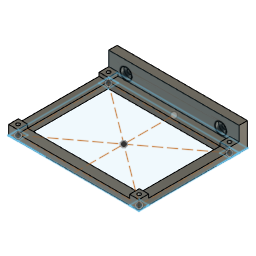
soporteSKR v3 (Autodesk Fusion 360 design; units mm, degrees)
Autodesk Fusion 360 part; units mm, degrees
sketch "Sketch7" plane through (0, 0, 0) normal (0, 0, 1) x (1, 0, 0)
  line L0 (9.0135, 7.5242) -> (118.6835, 7.5242)
  line L1 (118.6835, 7.5242) -> (118.6835, 98.8242)
  line L2 (118.6835, 98.8242) -> (9.0135, 98.8242)
  line L3 (9.0135, 98.8242) -> (9.0135, 7.5242)
  line L4 (63.8485, 7.5242) -> (63.8485, 91.8242) construction
  line L5 (118.6835, 91.8242) -> (9.0135, 91.8242)
  line L6 (12.9235, 11.6242) -> (114.7735, 11.6242) construction
  line L7 (114.7735, 11.6242) -> (114.7735, 87.7242) construction
  line L8 (114.7735, 87.7242) -> (12.9235, 87.7242) construction
  line L9 (12.9235, 87.7242) -> (12.9235, 11.6242) construction
  line L10 (12.9235, 11.6242) -> (114.7735, 87.7242) construction
  line L11 (114.7735, 11.6242) -> (12.9235, 87.7242) construction
  line L12 (9.0135, 91.8242) -> (16.8335, 91.8242)
  line L13 (16.8335, 91.8242) -> (16.8335, 83.6242)
  line L14 (16.8335, 83.6242) -> (9.0135, 83.6242)
  line L15 (9.0135, 83.6242) -> (9.0135, 91.8242)
  line L16 (9.0135, 91.8242) -> (16.8335, 83.6242) construction
  line L17 (16.8335, 91.8242) -> (9.0135, 83.6242) construction
  line L18 (9.0135, 7.5242) -> (16.8335, 7.5242)
  line L19 (16.8335, 7.5242) -> (16.8335, 15.7242)
  line L20 (16.8335, 15.7242) -> (9.0135, 15.7242)
  line L21 (9.0135, 15.7242) -> (9.0135, 7.5242)
  line L22 (9.0135, 7.5242) -> (16.8335, 15.7242) construction
  line L23 (16.8335, 7.5242) -> (9.0135, 15.7242) construction
  line L24 (118.6835, 7.5242) -> (110.8635, 7.5242)
  line L25 (110.8635, 7.5242) -> (110.8635, 15.7242)
  line L26 (110.8635, 15.7242) -> (118.6835, 15.7242)
  line L27 (118.6835, 15.7242) -> (118.6835, 7.5242)
  line L28 (118.6835, 7.5242) -> (110.8635, 15.7242) construction
  line L29 (110.8635, 7.5242) -> (118.6835, 15.7242) construction
  line L30 (118.6835, 91.8242) -> (110.8635, 91.8242)
  line L31 (110.8635, 91.8242) -> (110.8635, 83.6242)
  line L32 (110.8635, 83.6242) -> (118.6835, 83.6242)
  line L33 (118.6835, 83.6242) -> (118.6835, 91.8242)
  line L34 (118.6835, 91.8242) -> (110.8635, 83.6242) construction
  line L35 (110.8635, 91.8242) -> (118.6835, 83.6242) construction
  circle A0 centre (12.9235, 87.7242) radius 1.5
  circle A1 centre (114.7735, 87.7242) radius 1.5
  circle A2 centre (12.9235, 11.6242) radius 1.5
  circle A3 centre (114.7735, 11.6242) radius 1.5
  point P0 (63.8485, 49.6742)
  point P1 (12.9235, 87.7242)
  point P2 (12.9235, 11.6242)
  point P3 (114.7735, 11.6242)
  point P4 (114.7735, 87.7242)
  dimension "d70" = 109.67
  dimension "d71" = 91.3
  dimension "d72" = 84.3
  dimension "d73" = 101.85
  dimension "d74" = 76.1
  dimension "d89" = 3
  dimension "d90" = 3
  dimension "d91" = 3
  dimension "d92" = 3
  constraint horizontal L0
  constraint vertical L1
  constraint horizontal L2
  constraint vertical L3
  constraint midpoint L0 L4.start
  constraint perpendicular L0 L4
  constraint coincident L1 L5.start
  constraint coincident L3 L5.end
  constraint perpendicular L3 L5
  constraint horizontal L6
  constraint perpendicular L6 L7
  constraint parallel L6 L8
  constraint parallel L7 L9
  constraint coincident L10 P0
  constraint coincident L11 P0
  constraint midpoint L4 P0
  constraint horizontal L12
  constraint perpendicular L12 L13
  constraint parallel L12 L14
  constraint parallel L13 L15
  constraint coincident L16 P1
  constraint coincident L17 P1
  constraint coincident P1 L8.end
  constraint horizontal L18
  constraint perpendicular L18 L19
  constraint parallel L18 L20
  constraint parallel L19 L21
  constraint coincident L22 P2
  constraint coincident L23 P2
  constraint coincident P2 L6.start
  constraint horizontal L24
  constraint perpendicular L24 L25
  constraint parallel L24 L26
  constraint parallel L25 L27
  constraint coincident L28 P3
  constraint coincident L29 P3
  constraint coincident P3 L6.end
  constraint horizontal L30
  constraint perpendicular L30 L31
  constraint parallel L30 L32
  constraint parallel L31 L33
  constraint coincident L34 P4
  constraint coincident L35 P4
  constraint coincident P4 L7.end
  measures "d70" distance of L0.start L0.end
  measures "d71" distance of L0.start L2.end
  measures "d72" distance of L4.start L4.end
  measures "d73" distance of P4 P1
  measures "d74" distance of P3 P4
  measures "d89" diameter of A0
  measures "d90" diameter of A1
  measures "d91" diameter of A2
  measures "d92" diameter of A3
extrude "Extrude11" add sketch "Sketch7" along normal blind 5 contours L0 L3 L18 L19 L20 L21 | L0 L1 L3 L5 L13 L14 L19 L20 L25 L26 L31 L32 | L0 L1 L24 L25 L26 L27 | L3 L5 L12 L13 L14 L15 | L1 L5 L30 L31 L32 L33 | A0 | A1 | A2 | A3
extrude "Extrude13" cut sketch "Sketch7" along normal blind 8 contours L0 L3 L18 L19 L20 L21 | L0 L1 L24 L25 L26 L27 | L3 L5 L12 L13 L14 L15 | L1 L5 L30 L31 L32 L33 | A0 | A1 | A2 | A3
extrude "Extrude14" add sketch "Sketch7" along normal blind 8 contours L0 L3 L18 L19 L20 L21 | L0 L1 L24 L25 L26 L27 | L3 L5 L12 L13 L14 L15 | L1 L5 L30 L31 L32 L33 | A0 | A1 | A2 | A3
extrude "Extrude15" add sketch "Sketch7" along normal blind 20 contours L1 L2 L3 L5 L12 L30
extrude "Extrude16" cut sketch "Sketch7" along normal blind 22 contours A0 | A1 | A2 | A3
hole "Hole8" at (103.6835, 91.8242, 14) at (24.0135, 91.8242, 14) direction (0, 1, 0) diameter 4 end through all
sketch "Sketch10" plane through (0, 0, 5) normal (0, 0, 1) x (-1, 0, 0)
  line L0 (-16.8335, -83.6242) -> (-9.0135, -83.6242)
  line L1 (-9.0135, -83.6242) -> (-9.0135, -15.7242)
  line L2 (-9.0135, -15.7242) -> (-16.8335, -15.7242)
  line L3 (-16.8335, -15.7242) -> (-16.8335, -7.5242)
  line L4 (-16.8335, -7.5242) -> (-110.8635, -7.5242)
  line L5 (-110.8635, -7.5242) -> (-110.8635, -15.7242)
  line L6 (-110.8635, -15.7242) -> (-118.6835, -15.7242)
  line L7 (-118.6835, -15.7242) -> (-118.6835, -83.6242)
  line L8 (-118.6835, -83.6242) -> (-110.8635, -83.6242)
  line L9 (-110.8635, -83.6242) -> (-110.8635, -91.8242)
  line L10 (-110.8635, -91.8242) -> (-16.8335, -91.8242)
  line L11 (-16.8335, -91.8242) -> (-16.8335, -83.6242)
  line L12 (-16.8335, -83.6242) -> (-110.8635, -83.6242)
  line L13 (-110.8635, -83.6242) -> (-110.8635, -15.7242)
  line L14 (-110.8635, -15.7242) -> (-16.8335, -15.7242)
  line L15 (-16.8335, -15.7242) -> (-16.8335, -83.6242)
  constraint horizontal L12
  constraint vertical L13
  constraint horizontal L14
  constraint vertical L15
  constraint coincident L5.end L6.start
  constraint coincident L0.start L11.end
extrude "Extrude17" cut sketch "Sketch10" against normal blind 29 contours L12 L13 L14 L15
move_face "MoveFace1" to x (1, 0, 0) y (0, 1, 0) z (0, 0, 1) at (0.1522, 0, -1.9942) 2 faces at (102.9066, 94.1575, 12.157) (24.2126, 94.1575, 12.0099)
move_face "MoveFace2" to x (1, 0, 0) y (0, 1, 0) z (0, 0, 1) at (-0.5834, 0, -1.913) 2 faces at (103.0588, 94.1575, 10.1628) (24.3648, 94.1575, 10.0157)
sketch "Sketch12" plane through (0, 91.8242, 0) normal (0, -1, 0) x (1, 0, 0)
  circle A0 centre (103.2523, 10.0928) radius 2
  circle A1 centre (23.5823, 10.0928) radius 2
  line L0 (9.0135, 8) -> (16.8335, 8)
  line L1 (16.8335, 8) -> (16.8335, 5)
  line L2 (16.8335, 5) -> (110.8635, 5)
  line L3 (110.8635, 5) -> (110.8635, 8)
  line L4 (110.8635, 8) -> (118.6835, 8)
  line L5 (118.6835, 8) -> (118.6835, 20)
  line L6 (118.6835, 20) -> (9.0135, 20)
  line L7 (9.0135, 20) -> (9.0135, 8)
  circle A2 centre (23.5823, 10.0928) radius 4.8
  circle A3 centre (103.2523, 10.0928) radius 4.8
  dimension "d102" = 2.8
  dimension "d105" = 2.8
extrude "Extrude19" cut sketch "Sketch12" against normal blind 3 contours A3
extrude "Extrude18" cut sketch "Sketch12" against normal blind 3 contours A2
